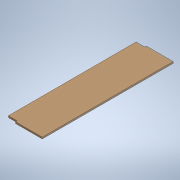
# Autodesk Inventor part: basedraws
Saved by Autodesk Inventor 2022 (Build 260153000, 153)
## iProperties
Created: 2022-02-21
Part Number: basedraws
Material: MDF Medium Density Fiberboard
Document SubType Name: Modeling
Designer: MarkP
Density: 0.8 g/cm^3
Appearance: Cardboard - Corrugated
Author: MarkP
Autodesk Inventor part; units mm, degrees
ref_plane "YZ Plane" through (0, 0, 0) normal (1, 0, 0) x (0, 1, 0)
ref_plane "XZ Plane" through (0, 0, 0) normal (0, 1, 0) x (-1, 0, 0)
ref_plane "XY Plane" through (0, 0, 0) normal (0, 0, 1) x (1, 0, 0)
sketch "Sketch1" plane through (0, 0, 0) normal (0, 1, 0) x (-1, 0, 0)
  line L0 (0, 0) -> (400, 0)
  line L1 (400, 0) -> (400, -1476)
  line L2 (400, -1476) -> (0, -1476)
  line L3 (0, -1476) -> (0, 0)
  line L4 (400, -1476) -> (418, -1476)
  line L5 (400, -1476) -> (300, -1476)
  line L6 (300, -1476) -> (300, -1458)
  line L7 (300, -1458) -> (400, -1458)
  line L8 (400, -1458) -> (400, -1476)
  line L9 (400, 0) -> (300, 0)
  line L10 (300, 0) -> (300, -18)
  line L11 (300, -18) -> (400, -18)
  line L12 (400, -18) -> (400, 0)
  dimension "d0" = 400
  dimension "d1" = 1476
  dimension "d4" = 100
  dimension "d5" = 18
  dimension "d6" = 100
  dimension "d7" = 18
  constraints: 26 end point, 6 parallel, 4 horizontal, 3 perpendicular
  measures "d0" distance of L1.end L2.end
  measures "d1" distance of L0.end L1.end
  measures "d4" distance of L6.end L7.end
  measures "d5" distance of L5.end L6.end
  measures "d6" distance of L11.end L10.end
  measures "d7" distance of L10.end L9.end
extrude "Extrusion1" add sketch "Sketch1" along normal blind 18 contours L0 L10 L11 L1 L7 L6 L2 L3
sketch "Sketch2" plane through (-300, 0, 0) normal (0, 0, 1) x (1, 0, 0)
  circle A0 centre (150, 9) radius 2.5
  circle A1 centre (0, 9) radius 2.5
  point P0 (300, 0)
  dimension "d13" = 5
  dimension "d14" = 5
  constraints: 2 centre point
  measures "d13" diameter of A0
  measures "d14" diameter of A1
sketch "Sketch3" plane through (0, 0, -1476) normal (0, 0, -1) x (-1, 0, 0)
  line L0 (300, 0) -> (300, 18) projected
  circle A0 centre (150, 9) radius 2.5
  circle A1 centre (300, 9) radius 2.5
  dimension "d18" = 5
  dimension "d19" = 5
  constraints: 2 centre point
  measures "d18" diameter of A0
  measures "d19" diameter of A1
extrude "Extrusion2" cut sketch "Sketch3" against normal blind 32
extrude "Extrusion3" cut sketch "Sketch2" against normal blind 32
body "Solid1"
